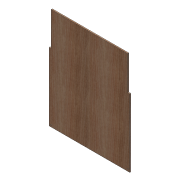
# Autodesk Inventor part: ElectronicsBoard
Saved by Autodesk Inventor 2012 (Build 160160000, 160)
## iProperties
Created: 2012-11-22
Part Number: ElectronicsBoard
Material: Wood (Birch)
Document SubType Name: Modeling
Designer: JesseK
Mass: 1081.33 g
Surface Area: 6336.74 cm^2
Volume: 1966.05 cm^3
Density: 0.55 g/cm^3
Author: JesseK
Autodesk Inventor part; units mm, degrees
ref_plane "YZ Plane" through (0, 0, 0) normal (1, 0, 0) x (0, 1, 0)
ref_plane "XZ Plane" through (0, 0, 0) normal (0, 1, 0) x (-1, 0, 0)
ref_plane "XY Plane" through (0, 0, 0) normal (0, 0, 1) x (1, 0, 0)
sketch "Sketch1" plane through (0, 0, 0) normal (0, 0, 1) x (1, 0, 0)
  line L0 (0, 0) -> (482.6, 0)
  line L1 (482.6, 0) -> (482.6, 558.8)
  line L2 (482.6, 558.8) -> (0, 558.8)
  line L3 (0, 558.8) -> (0, 0)
  circle A0 centre (12.7, 12.7) radius 3.175
  circle A1 centre (469.9, 12.7) radius 3.175
  dimension "d0" = 558.8
  dimension "d1" = 482.6
  dimension "d2" = 6.35
  dimension "d3" = 6.35
  dimension "d4" = 12.7
  dimension "d5" = 12.7
  dimension "d7" = 12.7
  dimension "d8" = 12.7
  constraints: 8 end point, 2 centre point, 2 parallel, 1 horizontal, 1 perpendicular
  measures "d0" distance of L2.end L0.start
  measures "d1" distance of L1.end L2.end
  measures "d2" diameter of A0
  measures "d3" diameter of A1
  measures "d4" distance from line of L0 A0.centre
  measures "d5" distance from line of L0 A1.centre
  measures "d7" distance from line of L1 A1.centre
  measures "d8" distance from line of L3 A0.centre
extrude "Extrusion1" add sketch "Sketch1" along normal blind 6.35
sketch "Sketch2" plane through (0, 0, 0) normal (0, 0, -1) x (-1, 0, 0)
  line L0 (0, 558.8) -> (0, 0) projected
  line L1 (-482.6, 558.8) -> (0, 558.8) projected
  line L2 (-482.6, 0) -> (-482.6, 558.8) projected
  line L3 (-482.6, 558.8) -> (-457.2, 558.8)
  line L4 (-457.2, 558.8) -> (-457.2, 406.4)
  line L5 (-457.2, 406.4) -> (-482.6, 406.4)
  line L6 (-482.6, 406.4) -> (-482.6, 558.8)
  line L7 (0, 558.8) -> (-25.4, 558.8)
  line L8 (-25.4, 558.8) -> (-25.4, 406.4)
  line L9 (-25.4, 406.4) -> (0, 406.4)
  line L10 (0, 406.4) -> (0, 558.8)
  dimension "d13" = 25.4
  dimension "d16" = 152.4
  constraints: 16 end point, 4 parallel, 2 collinear, 2 equal length, 2 horizontal, 2 perpendicular, 2 point on line
  measures "d13" distance of L3.start L3.end
  measures "d16" distance between parallel lines of L1 L5
extrude "Extrusion2" cut sketch "Sketch2" against normal through all
sketch "Sketch3" plane through (0, 0, 6.35) normal (0, 0, 1) x (1, 0, 0)
  line L0 (457.2, 406.4) -> (457.2, 558.8) projected
  line L1 (25.4, 558.8) -> (457.2, 558.8) projected
  line L2 (25.4, 558.8) -> (25.4, 406.4) projected
  circle A0 centre (38.1, 546.1) radius 3.175
  circle A1 centre (444.5, 546.1) radius 3.175
  dimension "d17" = 6.35
  dimension "d18" = 6.35
  dimension "d19" = 12.7
  dimension "d20" = 12.7
  dimension "d21" = 12.7
  dimension "d22" = 12.7
  constraints: 2 centre point
  measures "d17" diameter of A1
  measures "d18" diameter of A0
  measures "d19" distance from line of L1 A0.centre
  measures "d20" distance from line of L2 A0.centre
  measures "d21" distance from line of L0 A1.centre
  measures "d22" distance from line of L1 A1.centre
extrude "Extrusion3" cut sketch "Sketch3" against normal through all
body "Solid1"
